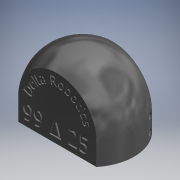
# Autodesk Inventor part: Wheel cover Alpha
Saved by Autodesk Inventor 2019 (Build 230136000, 136)
## iProperties
Part Number: Wheel cover Alpha
Material: Generic
Document SubType Name: Modeling
Designer: Delta
Appearance: Default
Author: Delta
Autodesk Inventor part; units mm, degrees
ref_plane "YZ Plane" through (0, 0, 0) normal (1, 0, 0) x (0, 1, 0)
ref_plane "XZ Plane" through (0, 0, 0) normal (0, 1, 0) x (-1, 0, 0)
ref_plane "XY Plane" through (0, 0, 0) normal (0, 0, 1) x (1, 0, 0)
sketch "Sketch1" plane through (0, 0, 0) normal (0, 0, 1) x (1, 0, 0)
  circle A0 centre (0, 0) radius 41.275
  circle A1 centre (0, 0) radius 44.45
  line L0 (-44.45, 0) -> (-41.275, 0)
  line L1 (41.275, 0) -> (44.45, 0)
  line L2 (-44.45, 0) -> (-41.275, 0)
  line L3 (-41.275, 0) -> (-41.275, -25.4)
  line L4 (-41.275, -25.4) -> (-44.45, -25.4)
  line L5 (-44.45, -25.4) -> (-44.45, 0)
  line L6 (41.275, 0) -> (44.45, 0)
  line L7 (44.45, 0) -> (44.45, -25.4)
  line L8 (44.45, -25.4) -> (41.275, -25.4)
  line L9 (41.275, -25.4) -> (41.275, 0)
  dimension "d0" = 82.55
  dimension "d1" = 88.9
  dimension "d2" = 25.4
  dimension "d3" = 25.4
  constraints: 20 end point, 4 parallel, 4 point on circle, 3 horizontal, 2 centre point, 2 coincident, 2 perpendicular, 2 point on line
  measures "d0" diameter of A0
  measures "d1" diameter of A1
  measures "d2" distance of L2.end L3.end
  measures "d3" distance of L6.end L7.end
extrude "Extrusion1" add sketch "Sketch1" along normal blind 59.69 contours A0 L0 A1 L1 | L1 A1 L9 | L3 A1 L0 | L7 L8 L9 A1 | A1 L3 L4 L5
sketch "Sketch2" plane through (0, 0, 59.69) normal (0, 0, 1) x (1, 0, 0)
  line L0 (-44.45, -25.4) -> (-41.275, -25.4) projected
  arc A0 (44.45, 0) -> (-44.45, 0) centre (0, 0) ccw projected
  line L1 (-44.45, -25.4) -> (44.45, -25.4)
  line L2 (44.45, -25.4) -> (44.45, 0)
  line L3 (44.45, 0) -> (-44.45, 0)
  line L4 (-44.45, 0) -> (-44.45, -25.4)
  line L5 (44.45, -25.4) -> (44.45, 0) projected
  arc A1 (44.45, 0) -> (-44.45, 0) centre (0, 0) ccw
  constraints: 8 end point, 2 parallel, 2 point on circle, 1 centre point, 1 horizontal, 1 perpendicular, 1 tangent
extrude "Extrusion2" add sketch "Sketch2" along normal blind 3.175
sketch "Sketch3" plane through (41.275, -25.4, 0) normal (-1, 0, 0) x (0, 0, 1)
  line L0 (0, 0) -> (59.69, 0) projected
  line L1 (0, 0) -> (12.7, 0)
  line L2 (12.7, 0) -> (12.7, 25.4)
  line L3 (12.7, 25.4) -> (0, 25.4)
  line L4 (0, 25.4) -> (0, 0)
  dimension "d8" = 12.7
  dimension "d9" = 25.4
  constraints: 8 end point, 2 parallel, 1 horizontal, 1 perpendicular
  measures "d8" distance of L3.end L2.end
  measures "d9" distance of L2.end L1.end
extrude "Extrusion3" add sketch "Sketch3" along normal blind 9.525
ref_plane "Work Plane1" through (0, -25.4, 0) normal (-1, 0, 0) x (0, 0, 1)
mirror "Mirror1" about plane through (0, -25.4, 0) normal (-1, 0, 0) of "Extrusion3"
ref_plane "Work Plane2" through (41.275, 0, 0) normal (0, -1, 0) x (1, 0, 0)
sketch "Sketch5" plane through (41.275, 0, 0) normal (0, -1, 0) x (1, 0, 0)
  line L0 (-85.725, 0) -> (-85.725, 62.865) projected
  line L1 (-85.725, 0) -> (-85.725, 62.865)
  arc A0 (-85.725, 62.865) -> (-85.725, 0) centre (-47.625, 31.4325) ccw
  line L2 (-41.275, 62.865) -> (-41.275, -18.3182)
  line L3 (3.175, 0) -> (3.175, 62.865) projected
  dimension "d12" = 44.45
  dimension "d13" = 44.45
  dimension "d33" = 38.1
  constraints: 4 end point, 2 point on circle, 2 vertical, 1 centre point
  measures "d12" distance between parallel lines of L3 L2
  measures "d13" distance between parallel lines of L0 L2
  measures "d33" distance from line of L0 A0.centre
revolve "Revolution1" add sketch "Sketch5" angle 180 about axis through (0, 0, 62.865) along (0, 0, -1)
sketch "Sketch6" plane through (6.35, 0, 31.4325) normal (0, -1, 0) x (1, 0, 0)
  line L0 (38.1, -31.4325) -> (38.1, 31.4325) projected
  line L1 (38.1, -31.4325) -> (38.1, 31.4325)
  arc A0 (38.1, -31.4325) -> (38.1, 31.4325) centre (0, 0) ccw projected
  line L2 (38.1, -31.4325) -> (38.1, 31.4325) projected
  arc A1 (38.1, -31.4325) -> (38.1, 31.4325) centre (0, 0) ccw
  point P0 (-6.35, -31.4325)
  constraints: 2 end point, 2 point on circle, 1 centre point, 1 collinear, 1 concentric
extrude "Extrusion4" add sketch "Sketch6" along normal blind 25.4
ref_plane "Work Plane3" through (0, -25.4, 0) normal (1, 0, 0) x (0, 0, -1)
mirror "Mirror2" about plane through (0, -25.4, 0) normal (1, 0, 0) of "Extrusion4"
sketch "Sketch7" plane through (31.75, -25.4, 0) normal (-1, 0, 0) x (0, 0, 1)
  line L0 (12.7, 0) -> (12.7, 25.4) projected
  line L1 (0, 25.4) -> (0, 0) projected
  line L2 (0, 0) -> (12.7, 0) projected
  circle A0 centre (6.35, 24.003) radius 1.524
  circle A1 centre (6.35, 8.001) radius 1.524
  dimension "d18" = 6.35
  dimension "d19" = 6.35
  dimension "d20" = 8.001
  dimension "d21" = 24.003
  dimension "d22" = 6.35
  dimension "d25" = 3.048
  dimension "d26" = 3.048
  constraints: 2 centre point, 2 coincident
  measures "d18" distance from line of L0 point (6.35, 8.001)
  measures "d19" distance from line of L1 point (6.35, 8.001)
  measures "d20" distance from line of L2 point (6.35, 8.001)
  measures "d21" distance from line of point (6.35, 24.003) L2
  measures "d22" distance from line of L0 point (6.35, 24.003)
  measures "d25" diameter of A0
  measures "d26" diameter of A1
sketch "Sketch8" plane through (31.75, 0, 0) normal (0, 1, 0) x (1, 0, 0)
  line L0 (9.525, -12.7) -> (9.525, -59.69) projected
  line L1 (0, -12.7) -> (0, 0) projected
  line L2 (9.525, -12.7) -> (0, -12.7)
  line L3 (0, -12.7) -> (0, 0)
  line L4 (0, 0) -> (9.525, 0)
  line L5 (9.525, 0) -> (9.525, -12.7)
  point P0 (-31.75, 0)
  constraints: 8 end point, 2 parallel, 1 horizontal, 1 perpendicular
extrude "Extrusion5" add sketch "Sketch8" along normal blind 2.54
extrude "Extrusion6" cut sketch "Sketch7" against normal through all
ref_plane "Work Plane4" through (55.7424, 0, 31.4325) normal (-1, 0, 0) x (0, -1, 0)
sketch "Sketch9" plane through (55.7424, 0, 31.4325) normal (-1, 0, 0) x (0, -1, 0)
  circle A0 centre (17.399, -25.0825) radius 1.524 projected
  circle A1 centre (17.399, -25.0825) radius 3.175
  circle A2 centre (1.397, -25.0825) radius 1.524 projected
  circle A3 centre (1.397, -25.0825) radius 3.175
  point P0 (0, -31.4325)
  dimension "d29" = 6.35
  dimension "d30" = 6.35
  constraints: 2 centre point, 2 coincident
  measures "d29" diameter of A1
  measures "d30" diameter of A3
extrude "Extrusion7" cut sketch "Sketch9" along normal blind 19.05
ref_plane "Work Plane5" through (0, -25.4, 0) normal (1, 0, 0) x (0, 0, -1)
mirror "Mirror3" about plane through (0, -25.4, 0) normal (1, 0, 0) of "Extrusion7", "Extrusion6", "Extrusion5"
sketch "Sketch10" plane through (0, 0, 59.69) normal (0, 0, -1) x (-1, 0, 0)
  line L0 (-11.0899, 12.4283) -> (34.7993, 12.4283) construction
  line L1 (34.7993, 12.4283) -> (34.7993, -9.7515) construction
  line L2 (34.7993, -9.7515) -> (-11.0899, -9.7515) construction
  line L3 (-11.0899, -9.7515) -> (-11.0899, 12.4283) construction
  line L4 (-4.0812, -3.8275) -> (-7.6627, -12.2101)
  line L5 (-7.6627, -12.2101) -> (-9.5307, -12.2101)
  line L6 (-9.5307, -12.2101) -> (-7.2768, -3.8275)
  line L7 (-7.2768, -3.8275) -> (-4.0812, -3.8275)
  line L8 (-4.9303, 3.1812) -> (-7.9869, 3.1812)
  line L9 (-7.9869, 3.1812) -> (-7.9869, 6.8245)
  line L10 (-7.9869, 6.8245) -> (-4.9303, 6.8245)
  line L11 (-4.9303, 6.8245) -> (-4.9303, 3.1812)
  spline S0 degree 2 poles (6.8332, -0.1533) (6.8332, -4.1053) (4.3014, -10.0951) (2.0629, -12.735) knots 0 0 0 1 2 2 2
  line L12 (2.0629, -12.735) -> (-0.8702, -12.735)
  line L13 (-0.8702, -12.735) -> (-0.8702, -12.6115)
  spline S1 degree 2 poles (-0.8702, -12.6115) (0.1178, -11.7315) (2.1093, -9.1534) (2.8503, -7.6097) knots 0 0 0 1 2 2 2
  spline S2 degree 2 poles (2.8503, -7.6097) (3.653, -5.9579) (4.5793, -2.2837) (4.5793, -0.1533) knots 0 0 0 1 2 2 2
  spline S3 degree 2 poles (4.5793, -0.1533) (4.5793, 1.9616) (3.6376, 5.713) (2.8503, 7.303) knots 0 0 0 1 2 2 2
  spline S4 degree 2 poles (2.8503, 7.303) (2.0784, 8.8931) (0.1024, 11.4249) (-0.8702, 12.3048) knots 0 0 0 1 2 2 2
  line L14 (-0.8702, 12.3048) -> (-0.8702, 12.4283)
  line L15 (-0.8702, 12.4283) -> (2.0629, 12.4283)
  spline S5 degree 2 poles (2.0629, 12.4283) (4.286, 9.7885) (6.8332, 3.8296) (6.8332, -0.1533) knots 0 0 0 1 2 2 2
  point P0 (0, 0)
  constraints: 2 other
extrude "Extrusion8" cut sketch "Sketch10" against normal blind 1.27
sketch "Sketch11" plane through (0, 0, 62.865) normal (0, 0, 1) x (1, 0, 0)
  line L0 (-39.7477, -3.175) -> (39.7477, -3.175) construction
  line L1 (39.7477, -3.175) -> (39.7477, -22.225) construction
  line L2 (39.7477, -22.225) -> (-39.7477, -22.225) construction
  line L3 (-39.7477, -22.225) -> (-39.7477, -3.175) construction
  line L4 (-42.9227, -25.4) -> (-42.9227, 0) projected
  line L5 (42.9227, 0) -> (42.9227, -25.4) projected
  line L6 (-44.45, -25.4) -> (44.45, -25.4) projected
  arc A0 (42.9227, 0) -> (-42.9227, 0) centre (0, 0) ccw projected
  line L7 (42.9227, -25.4) -> (42.9227, 0) projected
  line L8 (-42.9227, 0) -> (42.9227, 0)
  line L9 (0, 0) -> (0, 42.9227)
  arc A1 (30.2227, 0) -> (-30.2227, 0) centre (0, 0) ccw
  spline S0 degree 2 poles (-39.0273, -8.6682) (-39.0273, -7.4461) (-38.2297, -5.4135) (-37.535, -4.6802) knots 0 0 0 1 2 2 2
  spline S1 degree 2 poles (-37.535, -4.6802) (-36.8789, -3.9726) (-34.9621, -3.1879) (-33.9844, -3.1879) knots 0 0 0 1 2 2 2
  spline S2 degree 2 poles (-33.9844, -3.1879) (-32.8909, -3.1879) (-31.1155, -3.9212) (-30.4594, -4.6158) knots 0 0 0 1 2 2 2
  spline S3 degree 2 poles (-30.4594, -4.6158) (-29.6361, -5.4906) (-28.7356, -8.3209) (-28.7356, -10.495) knots 0 0 0 1 2 2 2
  spline S4 degree 2 poles (-28.7356, -10.495) (-28.7356, -12.4633) (-29.6232, -15.9882) (-30.4852, -17.1589) knots 0 0 0 1 2 2 2
  spline S5 degree 2 poles (-30.4852, -17.1589) (-31.3986, -18.3939) (-33.9715, -19.6932) (-35.8497, -19.6932) knots 0 0 0 1 2 2 2
  spline S6 degree 2 poles (-35.8497, -19.6932) (-36.2743, -19.6932) (-37.2391, -19.6032) (-37.6508, -19.4745) knots 0 0 0 1 2 2 2
  line L10 (-37.6508, -19.4745) -> (-37.6508, -17.4291)
  line L11 (-37.6508, -17.4291) -> (-37.5479, -17.4291)
  spline S7 degree 2 poles (-37.5479, -17.4291) (-37.2777, -17.5834) (-36.1456, -17.8536) (-35.5667, -17.8536) knots 0 0 0 1 2 2 2
  spline S8 degree 2 poles (-35.5667, -17.8536) (-33.4826, -17.8536) (-31.1027, -15.1005) (-30.9354, -12.5533) knots 0 0 0 1 2 2 2
  spline S9 degree 2 poles (-30.9354, -12.5533) (-31.7845, -13.1323) (-33.3283, -13.6597) (-34.2417, -13.6597) knots 0 0 0 1 2 2 2
  spline S10 degree 2 poles (-34.2417, -13.6597) (-35.1164, -13.6597) (-36.5702, -13.2738) (-37.3034, -12.7206) knots 0 0 0 1 2 2 2
  spline S11 degree 2 poles (-37.3034, -12.7206) (-38.1525, -12.0645) (-39.0273, -10.0705) (-39.0273, -8.6682) knots 0 0 0 1 2 2 2
  spline S12 degree 2 poles (-30.884, -10.019) (-30.884, -8.4109) (-31.4757, -6.3783) (-32.0032, -5.8251) knots 0 0 0 1 2 2 2
  spline S13 degree 2 poles (-32.0032, -5.8251) (-32.4663, -5.3105) (-33.4312, -4.9246) (-33.9972, -4.9246) knots 0 0 0 1 2 2 2
  spline S14 degree 2 poles (-33.9972, -4.9246) (-35.3094, -4.9246) (-36.866, -6.8028) (-36.866, -8.5782) knots 0 0 0 1 2 2 2
  spline S15 degree 2 poles (-36.866, -8.5782) (-36.866, -9.5816) (-36.3515, -10.8809) (-35.7854, -11.3441) knots 0 0 0 1 2 2 2
  spline S16 degree 2 poles (-35.7854, -11.3441) (-35.3737, -11.6785) (-34.3574, -11.8972) (-33.7657, -11.8972) knots 0 0 0 1 2 2 2
  spline S17 degree 2 poles (-33.7657, -11.8972) (-33.0838, -11.8972) (-31.5143, -11.4213) (-30.9226, -11.0224) knots 0 0 0 1 2 2 2
  spline S18 degree 2 poles (-30.9226, -11.0224) (-30.9097, -10.8681) (-30.884, -10.3406) (-30.884, -10.019) knots 0 0 0 1 2 2 2
  spline S19 degree 2 poles (-27.1146, -8.6682) (-27.1146, -7.4461) (-26.317, -5.4135) (-25.6223, -4.6802) knots 0 0 0 1 2 2 2
  spline S20 degree 2 poles (-25.6223, -4.6802) (-24.9662, -3.9726) (-23.0494, -3.1879) (-22.0717, -3.1879) knots 0 0 0 1 2 2 2
  spline S21 degree 2 poles (-22.0717, -3.1879) (-20.9782, -3.1879) (-19.2029, -3.9212) (-18.5468, -4.6158) knots 0 0 0 1 2 2 2
  spline S22 degree 2 poles (-18.5468, -4.6158) (-17.7234, -5.4906) (-16.8229, -8.3209) (-16.8229, -10.495) knots 0 0 0 1 2 2 2
  spline S23 degree 2 poles (-16.8229, -10.495) (-16.8229, -12.4633) (-17.7106, -15.9882) (-18.5725, -17.1589) knots 0 0 0 1 2 2 2
  spline S24 degree 2 poles (-18.5725, -17.1589) (-19.4859, -18.3939) (-22.0588, -19.6932) (-23.9371, -19.6932) knots 0 0 0 1 2 2 2
  spline S25 degree 2 poles (-23.9371, -19.6932) (-24.3616, -19.6932) (-25.3264, -19.6032) (-25.7381, -19.4745) knots 0 0 0 1 2 2 2
  line L12 (-25.7381, -19.4745) -> (-25.7381, -17.4291)
  line L13 (-25.7381, -17.4291) -> (-25.6352, -17.4291)
  spline S26 degree 2 poles (-25.6352, -17.4291) (-25.365, -17.5834) (-24.2329, -17.8536) (-23.654, -17.8536) knots 0 0 0 1 2 2 2
  spline S27 degree 2 poles (-23.654, -17.8536) (-21.57, -17.8536) (-19.19, -15.1005) (-19.0227, -12.5533) knots 0 0 0 1 2 2 2
  spline S28 degree 2 poles (-19.0227, -12.5533) (-19.8718, -13.1323) (-21.4156, -13.6597) (-22.329, -13.6597) knots 0 0 0 1 2 2 2
  spline S29 degree 2 poles (-22.329, -13.6597) (-23.2038, -13.6597) (-24.6575, -13.2738) (-25.3908, -12.7206) knots 0 0 0 1 2 2 2
  spline S30 degree 2 poles (-25.3908, -12.7206) (-26.2398, -12.0645) (-27.1146, -10.0705) (-27.1146, -8.6682) knots 0 0 0 1 2 2 2
  spline S31 degree 2 poles (-18.9713, -10.019) (-18.9713, -8.4109) (-19.5631, -6.3783) (-20.0905, -5.8251) knots 0 0 0 1 2 2 2
  spline S32 degree 2 poles (-20.0905, -5.8251) (-20.5536, -5.3105) (-21.5185, -4.9246) (-22.0845, -4.9246) knots 0 0 0 1 2 2 2
  spline S33 degree 2 poles (-22.0845, -4.9246) (-23.3967, -4.9246) (-24.9534, -6.8028) (-24.9534, -8.5782) knots 0 0 0 1 2 2 2
  spline S34 degree 2 poles (-24.9534, -8.5782) (-24.9534, -9.5816) (-24.4388, -10.8809) (-23.8727, -11.3441) knots 0 0 0 1 2 2 2
  spline S35 degree 2 poles (-23.8727, -11.3441) (-23.4611, -11.6785) (-22.4448, -11.8972) (-21.853, -11.8972) knots 0 0 0 1 2 2 2
  spline S36 degree 2 poles (-21.853, -11.8972) (-21.1711, -11.8972) (-19.6017, -11.4213) (-19.0099, -11.0224) knots 0 0 0 1 2 2 2
  spline S37 degree 2 poles (-19.0099, -11.0224) (-18.997, -10.8681) (-18.9713, -10.3406) (-18.9713, -10.019) knots 0 0 0 1 2 2 2
  line L14 (4.5196, -19.3845) -> (-9.207, -19.3845)
  line L15 (-9.207, -19.3845) -> (-3.6495, -3.5095)
  line L16 (-3.6495, -3.5095) -> (-1.0379, -3.5095)
  line L17 (-1.0379, -3.5095) -> (4.5196, -19.3845)
  line L18 (1.6765, -17.5577) -> (-2.4016, -5.5936)
  line L19 (-2.4016, -5.5936) -> (-6.454, -17.5577)
  line L20 (-6.454, -17.5577) -> (1.6765, -17.5577)
  line L21 (22.3886, -19.3845) -> (12.5986, -19.3845)
  line L22 (12.5986, -19.3845) -> (12.5986, -17.1332)
  spline S38 degree 2 poles (12.5986, -17.1332) (13.6535, -16.1426) (15.5317, -14.3029) (16.4323, -13.3124) knots 0 0 0 1 2 2 2
  spline S39 degree 2 poles (16.4323, -13.3124) (18.2462, -11.3183) (19.5713, -8.9255) (19.5713, -7.6519) knots 0 0 0 1 2 2 2
  spline S40 degree 2 poles (19.5713, -7.6519) (19.5713, -6.9829) (19.1596, -5.9795) (18.7865, -5.6579) knots 0 0 0 1 2 2 2
  spline S41 degree 2 poles (18.7865, -5.6579) (18.4134, -5.3363) (17.4357, -5.0146) (16.8439, -5.0146) knots 0 0 0 1 2 2 2
  spline S42 degree 2 poles (16.8439, -5.0146) (16.2779, -5.0146) (15.1201, -5.2977) (14.5926, -5.5164) knots 0 0 0 1 2 2 2
  spline S43 degree 2 poles (14.5926, -5.5164) (14.1424, -5.6965) (13.3062, -6.2111) (13.0489, -6.3912) knots 0 0 0 1 2 2 2
  line L23 (13.0489, -6.3912) -> (12.9331, -6.3912)
  line L24 (12.9331, -6.3912) -> (12.9331, -4.127)
  spline S44 degree 2 poles (12.9331, -4.127) (13.5892, -3.8054) (15.9434, -3.175) (16.9983, -3.175) knots 0 0 0 1 2 2 2
  spline S45 degree 2 poles (16.9983, -3.175) (19.2239, -3.175) (21.7325, -5.5292) (21.7325, -7.5361) knots 0 0 0 1 2 2 2
  spline S46 degree 2 poles (21.7325, -7.5361) (21.7325, -8.4752) (21.2951, -10.0447) (20.9092, -10.7137) knots 0 0 0 1 2 2 2
  spline S47 degree 2 poles (20.9092, -10.7137) (20.5232, -11.4084) (19.404, -12.772) (18.7865, -13.4281) knots 0 0 0 1 2 2 2
  spline S48 degree 2 poles (18.7865, -13.4281) (17.7831, -14.5216) (15.3259, -16.863) (14.5926, -17.5448) knots 0 0 0 1 2 2 2
  line L25 (14.5926, -17.5448) -> (22.3886, -17.5448)
  line L26 (22.3886, -17.5448) -> (22.3886, -19.3845)
  spline S49 degree 2 poles (34.1341, -14.3415) (34.1341, -15.4865) (33.4008, -17.4419) (32.7318, -18.1623) knots 0 0 0 1 2 2 2
  spline S50 degree 2 poles (32.7318, -18.1623) (32.0628, -18.8828) (30.0688, -19.719) (28.8338, -19.719) knots 0 0 0 1 2 2 2
  spline S51 degree 2 poles (28.8338, -19.719) (27.7017, -19.719) (25.489, -19.2172) (24.6785, -18.8184) knots 0 0 0 1 2 2 2
  line L27 (24.6785, -18.8184) -> (24.6785, -16.5671)
  line L28 (24.6785, -16.5671) -> (24.8329, -16.5671)
  spline S52 degree 2 poles (24.8329, -16.5671) (25.0773, -16.7472) (25.9907, -17.2104) (26.5439, -17.4162) knots 0 0 0 1 2 2 2
  spline S53 degree 2 poles (26.5439, -17.4162) (27.1743, -17.6349) (28.2163, -17.8793) (28.8724, -17.8793) knots 0 0 0 1 2 2 2
  spline S54 degree 2 poles (28.8724, -17.8793) (29.5156, -17.8793) (30.7249, -17.4162) (31.1623, -16.9145) knots 0 0 0 1 2 2 2
  spline S55 degree 2 poles (31.1623, -16.9145) (31.5611, -16.4385) (31.9728, -15.1777) (31.9728, -14.3287) knots 0 0 0 1 2 2 2
  spline S56 degree 2 poles (31.9728, -14.3287) (31.9728, -13.4796) (31.5097, -12.399) (31.0723, -12.0388) knots 0 0 0 1 2 2 2
  spline S57 degree 2 poles (31.0723, -12.0388) (30.622, -11.64) (29.2841, -11.3055) (28.4736, -11.3055) knots 0 0 0 1 2 2 2
  spline S58 degree 2 poles (28.4736, -11.3055) (27.5988, -11.3055) (25.8621, -11.5756) (25.3346, -11.6914) knots 0 0 0 1 2 2 2
  line L29 (25.3346, -11.6914) -> (25.3346, -3.5095)
  line L30 (25.3346, -3.5095) -> (34.044, -3.5095)
  line L31 (34.044, -3.5095) -> (34.044, -5.3749)
  line L32 (34.044, -5.3749) -> (27.3801, -5.3749)
  line L33 (27.3801, -5.3749) -> (27.3801, -9.6073)
  spline S59 degree 2 poles (27.3801, -9.6073) (27.766, -9.5559) (28.5122, -9.5173) (28.8209, -9.5173) knots 0 0 0 1 2 2 2
  spline S60 degree 2 poles (28.8209, -9.5173) (30.0431, -9.5173) (31.7284, -9.9161) (32.5002, -10.5079) knots 0 0 0 1 2 2 2
  spline S61 degree 2 poles (32.5002, -10.5079) (33.285, -11.0996) (34.1341, -12.9007) (34.1341, -14.3415) knots 0 0 0 1 2 2 2
  spline S62 degree 2 poles (-31.9263, 14.8461) (-30.6882, 14.4351) (-29.0287, 12.7701) (-28.7516, 11.7429) knots 0 0 0 1 2 2 2
  spline S63 degree 2 poles (-28.7516, 11.7429) (-28.5479, 10.9108) (-28.7241, 9.3996) (-29.0889, 8.3008) knots 0 0 0 1 2 2 2
  line L34 (-29.0889, 8.3008) -> (-29.7794, 6.2202)
  line L35 (-29.7794, 6.2202) -> (-38.8195, 9.2207)
  line L36 (-38.8195, 9.2207) -> (-38.1362, 11.2793)
  spline S64 degree 2 poles (-38.1362, 11.2793) (-37.7131, 12.554) (-36.8508, 13.878) (-36.3436, 14.279) knots 0 0 0 1 2 2 2
  spline S65 degree 2 poles (-36.3436, 14.279) (-35.4755, 14.9587) (-33.2449, 15.2837) (-31.9263, 14.8461) knots 0 0 0 1 2 2 2
  spline S66 degree 2 poles (-32.3567, 13.5982) (-33.397, 13.9435) (-35.098, 13.7436) (-35.7417, 13.2009) knots 0 0 0 1 2 2 2
  spline S67 degree 2 poles (-35.7417, 13.2009) (-36.1879, 12.8122) (-36.8066, 11.8058) (-37.0765, 10.9926) knots 0 0 0 1 2 2 2
  line L37 (-37.0765, 10.9926) -> (-37.3804, 10.0769)
  line L38 (-37.3804, 10.0769) -> (-30.4209, 7.7669)
  line L39 (-30.4209, 7.7669) -> (-30.117, 8.6827)
  spline S68 degree 2 poles (-30.117, 8.6827) (-29.8519, 9.4812) (-29.7071, 10.775) (-29.8885, 11.3802) knots 0 0 0 1 2 2 2
  spline S69 degree 2 poles (-29.8885, 11.3802) (-30.1043, 12.1512) (-31.3018, 13.2481) (-32.3567, 13.5982) knots 0 0 0 1 2 2 2
  spline S70 degree 2 poles (-24.8557, 16.915) (-25.7947, 15.4816) (-28.4345, 14.9594) (-29.9195, 15.9322) knots 0 0 0 1 2 2 2
  spline S71 degree 2 poles (-29.9195, 15.9322) (-31.3787, 16.8881) (-32.1067, 19.5519) (-31.2988, 20.7852) knots 0 0 0 1 2 2 2
  spline S72 degree 2 poles (-31.2988, 20.7852) (-30.935, 21.3404) (-30.0496, 21.9877) (-29.5002, 22.0799) knots 0 0 0 1 2 2 2
  spline S73 degree 2 poles (-29.5002, 22.0799) (-28.9465, 22.1786) (-27.7344, 21.8736) (-27.0177, 21.4041) knots 0 0 0 1 2 2 2
  line L40 (-27.0177, 21.4041) -> (-26.4689, 21.0446)
  line L41 (-26.4689, 21.0446) -> (-29.1802, 16.9058)
  spline S74 degree 2 poles (-29.1802, 16.9058) (-28.1407, 16.2248) (-26.3513, 16.5475) (-25.7423, 17.4773) knots 0 0 0 1 2 2 2
  spline S75 degree 2 poles (-25.7423, 17.4773) (-25.5265, 17.8066) (-25.2563, 18.5431) (-25.2033, 18.8775) knots 0 0 0 1 2 2 2
  spline S76 degree 2 poles (-25.2033, 18.8775) (-25.1548, 19.2333) (-25.1355, 19.7558) (-25.1584, 19.9462) knots 0 0 0 1 2 2 2
  line L42 (-25.1584, 19.9462) -> (-25.1203, 20.0043)
  line L43 (-25.1203, 20.0043) -> (-24.0227, 19.2852)
  spline S77 degree 2 poles (-24.0227, 19.2852) (-24.0659, 19.0643) (-24.2061, 18.3995) (-24.2834, 18.1549) knots 0 0 0 1 2 2 2
  spline S78 degree 2 poles (-24.2834, 18.1549) (-24.3898, 17.8093) (-24.6188, 17.2765) (-24.8557, 16.915) knots 0 0 0 1 2 2 2
  spline S79 degree 2 poles (-27.8802, 20.5665) (-28.2954, 20.8201) (-28.9994, 21.0413) (-29.3053, 21.011) knots 0 0 0 1 2 2 2
  spline S80 degree 2 poles (-29.3053, 21.011) (-29.6455, 20.9847) (-30.2439, 20.5924) (-30.5104, 20.1856) knots 0 0 0 1 2 2 2
  spline S81 degree 2 poles (-30.5104, 20.1856) (-30.7726, 19.7853) (-30.9017, 19.0671) (-30.8216, 18.6824) knots 0 0 0 1 2 2 2
  spline S82 degree 2 poles (-30.8216, 18.6824) (-30.7307, 18.2999) (-30.3083, 17.691) (-29.9485, 17.4092) knots 0 0 0 1 2 2 2
  line L44 (-29.9485, 17.4092) -> (-27.8802, 20.5665)
  line L45 (-21.85, 20.8891) -> (-22.6646, 20.0023)
  line L46 (-22.6646, 20.0023) -> (-29.9918, 26.7332)
  line L47 (-29.9918, 26.7332) -> (-29.1772, 27.62)
  line L48 (-29.1772, 27.62) -> (-21.85, 20.8891)
  spline S83 degree 2 poles (-18.8752, 23.4407) (-19.6213, 22.8048) (-21.1874, 22.9405) (-21.9735, 23.8628) knots 0 0 0 1 2 2 2
  line L49 (-21.9735, 23.8628) -> (-24.5422, 26.8763)
  line L50 (-24.5422, 26.8763) -> (-25.159, 26.3506)
  line L51 (-25.159, 26.3506) -> (-25.8049, 27.1084)
  line L52 (-25.8049, 27.1084) -> (-25.1881, 27.6341)
  line L53 (-25.1881, 27.6341) -> (-26.5201, 29.1967)
  line L54 (-26.5201, 29.1967) -> (-25.6037, 29.9778)
  line L55 (-25.6037, 29.9778) -> (-24.2717, 28.4152)
  line L56 (-24.2717, 28.4152) -> (-22.5858, 29.8523)
  line L57 (-22.5858, 29.8523) -> (-21.9399, 29.0945)
  line L58 (-21.9399, 29.0945) -> (-23.6258, 27.6575)
  line L59 (-23.6258, 27.6575) -> (-21.4176, 25.0669)
  spline S84 degree 2 poles (-21.4176, 25.0669) (-21.0671, 24.6557) (-20.6522, 24.2284) (-20.3871, 24.1197) knots 0 0 0 1 2 2 2
  spline S85 degree 2 poles (-20.3871, 24.1197) (-20.1596, 24.0194) (-19.6443, 24.1645) (-19.3271, 24.4349) knots 0 0 0 1 2 2 2
  spline S86 degree 2 poles (-19.3271, 24.4349) (-19.1039, 24.6252) (-18.802, 25.1158) (-18.7431, 25.237) knots 0 0 0 1 2 2 2
  line L60 (-18.7431, 25.237) -> (-18.6902, 25.2821)
  line L61 (-18.6902, 25.2821) -> (-17.9892, 24.4597)
  spline S87 degree 2 poles (-17.9892, 24.4597) (-18.1876, 24.1689) (-18.6461, 23.636) (-18.8752, 23.4407) knots 0 0 0 1 2 2 2
  spline S88 degree 2 poles (-14.1689, 27.5855) (-14.2424, 27.4188) (-14.4792, 26.8384) (-14.6226, 26.6228) knots 0 0 0 1 2 2 2
  spline S89 degree 2 poles (-14.6226, 26.6228) (-14.8128, 26.3182) (-15.2403, 25.8687) (-15.7092, 25.6001) knots 0 0 0 1 2 2 2
  spline S90 degree 2 poles (-15.7092, 25.6001) (-16.0909, 25.3815) (-16.9458, 25.2743) (-17.3566, 25.3859) knots 0 0 0 1 2 2 2
  spline S91 degree 2 poles (-17.3566, 25.3859) (-17.7502, 25.4985) (-18.4813, 26.076) (-18.7192, 26.4912) knots 0 0 0 1 2 2 2
  spline S92 degree 2 poles (-18.7192, 26.4912) (-19.0875, 27.1342) (-19.0668, 28.3559) (-18.627, 28.9547) knots 0 0 0 1 2 2 2
  spline S93 degree 2 poles (-18.627, 28.9547) (-18.2427, 29.4951) (-16.9263, 30.4893) (-16.1293, 31.0081) knots 0 0 0 1 2 2 2
  line L62 (-16.1293, 31.0081) -> (-16.2444, 31.209)
  spline S94 degree 2 poles (-16.2444, 31.209) (-16.4516, 31.5707) (-16.9297, 31.8928) (-17.2035, 31.905) knots 0 0 0 1 2 2 2
  spline S95 degree 2 poles (-17.2035, 31.905) (-17.4773, 31.9171) (-18.0994, 31.6676) (-18.4075, 31.4911) knots 0 0 0 1 2 2 2
  spline S96 degree 2 poles (-18.4075, 31.4911) (-18.7692, 31.2839) (-19.6243, 30.5095) (-19.9943, 30.0218) knots 0 0 0 1 2 2 2
  line L63 (-19.9943, 30.0218) -> (-20.0546, 29.9872)
  line L64 (-20.0546, 29.9872) -> (-20.6646, 31.0522)
  spline S97 degree 2 poles (-20.6646, 31.0522) (-20.4226, 31.2975) (-19.4594, 32.1161) (-18.9302, 32.4192) knots 0 0 0 1 2 2 2
  spline S98 degree 2 poles (-18.9302, 32.4192) (-18.2873, 32.7875) (-17.2947, 33.0892) (-16.7968, 33.0275) knots 0 0 0 1 2 2 2
  spline S99 degree 2 poles (-16.7968, 33.0275) (-16.3095, 32.9686) (-15.5103, 32.35) (-15.1766, 31.7673) knots 0 0 0 1 2 2 2
  line L65 (-15.1766, 31.7673) -> (-12.748, 27.5276)
  line L66 (-12.748, 27.5276) -> (-13.7929, 26.9291)
  line L67 (-13.7929, 26.9291) -> (-14.1689, 27.5855)
  line L68 (-14.6676, 28.4562) -> (-15.6536, 30.1775)
  spline S100 degree 2 poles (-15.6536, 30.1775) (-16.0095, 29.9292) (-17.0762, 29.167) (-17.3698, 28.8565) knots 0 0 0 1 2 2 2
  spline S101 degree 2 poles (-17.3698, 28.8565) (-17.7122, 28.4913) (-17.9516, 27.6514) (-17.6831, 27.1826) knots 0 0 0 1 2 2 2
  spline S102 degree 2 poles (-17.6831, 27.1826) (-17.3761, 26.6468) (-16.4626, 26.4495) (-15.8866, 26.7795) knots 0 0 0 1 2 2 2
  spline S103 degree 2 poles (-15.8866, 26.7795) (-15.3976, 27.0595) (-14.8356, 27.9419) (-14.6676, 28.4562) knots 0 0 0 1 2 2 2
  line L69 (0.072, 30.5231) -> (-1.5565, 30.2968)
  line L70 (-1.5565, 30.2968) -> (-5.0598, 33.6364)
  line L71 (-5.0598, 33.6364) -> (-6.4971, 33.4366)
  line L72 (-6.4971, 33.4366) -> (-5.9755, 29.6828)
  line L73 (-5.9755, 29.6828) -> (-7.2293, 29.5086)
  line L74 (-7.2293, 29.5086) -> (-8.5403, 38.9429)
  line L75 (-8.5403, 38.9429) -> (-6.1091, 39.2807)
  spline S104 degree 2 poles (-6.1091, 39.2807) (-5.2987, 39.3934) (-4.1809, 39.3694) (-3.6394, 39.1174) knots 0 0 0 1 2 2 2
  spline S105 degree 2 poles (-3.6394, 39.1174) (-3.0978, 38.8653) (-2.3852, 37.9435) (-2.2822, 37.2019) knots 0 0 0 1 2 2 2
  spline S106 degree 2 poles (-2.2822, 37.2019) (-2.1388, 36.1697) (-2.9994, 34.624) (-3.8548, 34.1623) knots 0 0 0 1 2 2 2
  line L76 (-3.8548, 34.1623) -> (0.072, 30.5231)
  spline S107 degree 2 poles (-3.5757, 36.9208) (-3.6331, 37.3337) (-4.0118, 37.9279) (-4.3463, 38.0918) knots 0 0 0 1 2 2 2
  spline S108 degree 2 poles (-4.3463, 38.0918) (-4.6383, 38.2304) (-5.3695, 38.2769) (-5.8894, 38.2047) knots 0 0 0 1 2 2 2
  line L77 (-5.8894, 38.2047) -> (-7.1356, 38.0315)
  line L78 (-7.1356, 38.0315) -> (-6.6426, 34.4841)
  line L79 (-6.6426, 34.4841) -> (-5.5417, 34.637)
  spline S109 degree 2 poles (-5.5417, 34.637) (-4.9989, 34.7125) (-4.1615, 35.0237) (-3.9048, 35.3633) knots 0 0 0 1 2 2 2
  spline S110 degree 2 poles (-3.9048, 35.3633) (-3.6657, 35.6614) (-3.5077, 36.4315) (-3.5757, 36.9208) knots 0 0 0 1 2 2 2
  spline S111 degree 2 poles (6.9711, 33.2234) (6.768, 31.4287) (4.821, 29.6681) (3.3791, 29.8313) knots 0 0 0 1 2 2 2
  spline S112 degree 2 poles (3.3791, 29.8313) (1.8988, 29.9988) (0.432, 32.2077) (0.6281, 33.9411) knots 0 0 0 1 2 2 2
  spline S113 degree 2 poles (0.6281, 33.9411) (0.8294, 35.7205) (2.8012, 37.4938) (4.2278, 37.3324) knots 0 0 0 1 2 2 2
  spline S114 degree 2 poles (4.2278, 37.3324) (5.6697, 37.1693) (7.1733, 35.0105) (6.9711, 33.2234) knots 0 0 0 1 2 2 2
  spline S115 degree 2 poles (5.7362, 33.3631) (5.8924, 34.7437) (5.0396, 36.1996) (4.1115, 36.3046) knots 0 0 0 1 2 2 2
  spline S116 degree 2 poles (4.1115, 36.3046) (3.1835, 36.4096) (2.0192, 35.182) (1.863, 33.8014) knots 0 0 0 1 2 2 2
  spline S117 degree 2 poles (1.863, 33.8014) (1.7111, 32.4592) (2.5673, 30.964) (3.4954, 30.859) knots 0 0 0 1 2 2 2
  spline S118 degree 2 poles (3.4954, 30.859) (4.4158, 30.7549) (5.5818, 31.9979) (5.7362, 33.3631) knots 0 0 0 1 2 2 2
  spline S119 degree 2 poles (14.6415, 30.7601) (14.0424, 29.1135) (11.7156, 27.6848) (10.5115, 28.1229) knots 0 0 0 1 2 2 2
  spline S120 degree 2 poles (10.5115, 28.1229) (9.9675, 28.3209) (9.289, 28.8717) (8.9963, 29.241) knots 0 0 0 1 2 2 2
  line L80 (8.9963, 29.241) -> (8.8102, 28.9555)
  line L81 (8.8102, 28.9555) -> (7.7512, 29.3408)
  line L82 (7.7512, 29.3408) -> (11.1531, 38.6907)
  line L83 (11.1531, 38.6907) -> (12.2846, 38.279)
  line L84 (12.2846, 38.279) -> (11.0706, 34.9423)
  spline S121 degree 2 poles (11.0706, 34.9423) (11.6385, 35.1711) (12.8169, 35.3173) (13.448, 35.0877) knots 0 0 0 1 2 2 2
  spline S122 degree 2 poles (13.448, 35.0877) (14.5868, 34.6733) (15.23, 32.3776) (14.6415, 30.7601) knots 0 0 0 1 2 2 2
  spline S123 degree 2 poles (13.442, 31.0979) (13.8801, 32.302) (13.6014, 33.8162) (12.789, 34.1118) knots 0 0 0 1 2 2 2
  spline S124 degree 2 poles (12.789, 34.1118) (12.3321, 34.278) (11.2307, 34.1859) (10.7249, 33.9921) knots 0 0 0 1 2 2 2
  line L85 (10.7249, 33.9921) -> (9.3235, 30.1405)
  spline S125 degree 2 poles (9.3235, 30.1405) (9.6749, 29.7744) (10.2717, 29.3601) (10.6634, 29.2176) knots 0 0 0 1 2 2 2
  spline S126 degree 2 poles (10.6634, 29.2176) (11.5265, 28.9036) (12.9591, 29.7705) (13.442, 31.0979) knots 0 0 0 1 2 2 2
  spline S127 degree 2 poles (21.3296, 26.4091) (20.3319, 24.9035) (17.7969, 24.2221) (16.5873, 25.0237) knots 0 0 0 1 2 2 2
  spline S128 degree 2 poles (16.5873, 25.0237) (15.3455, 25.8466) (15.0449, 28.4811) (16.0085, 29.9353) knots 0 0 0 1 2 2 2
  spline S129 degree 2 poles (16.0085, 29.9353) (16.9977, 31.428) (19.5605, 32.1095) (20.7573, 31.3164) knots 0 0 0 1 2 2 2
  spline S130 degree 2 poles (20.7573, 31.3164) (21.9669, 30.5148) (22.3231, 27.9083) (21.3296, 26.4091) knots 0 0 0 1 2 2 2
  spline S131 degree 2 poles (20.2937, 27.0956) (21.0612, 28.2537) (20.9645, 29.9383) (20.1859, 30.4542) knots 0 0 0 1 2 2 2
  spline S132 degree 2 poles (20.1859, 30.4542) (19.4074, 30.9701) (17.8119, 30.407) (17.0444, 29.2488) knots 0 0 0 1 2 2 2
  spline S133 degree 2 poles (17.0444, 29.2488) (16.2983, 28.1228) (16.3801, 26.4018) (17.1586, 25.8859) knots 0 0 0 1 2 2 2
  spline S134 degree 2 poles (17.1586, 25.8859) (17.9307, 25.3742) (19.5348, 25.9503) (20.2937, 27.0956) knots 0 0 0 1 2 2 2
  spline S135 degree 2 poles (21.6452, 20.91) (20.9447, 21.5957) (20.9388, 23.1676) (21.7865, 24.0336) knots 0 0 0 1 2 2 2
  line L86 (21.7865, 24.0336) -> (24.5564, 26.8634)
  line L87 (24.5564, 26.8634) -> (23.9772, 27.4303)
  line L88 (23.9772, 27.4303) -> (24.6737, 28.1419)
  line L89 (24.6737, 28.1419) -> (25.2529, 27.5749)
  line L90 (25.2529, 27.5749) -> (26.6892, 29.0422)
  line L91 (26.6892, 29.0422) -> (27.5497, 28.1999)
  line L92 (27.5497, 28.1999) -> (26.1134, 26.7326)
  line L93 (26.1134, 26.7326) -> (27.6965, 25.183)
  line L94 (27.6965, 25.183) -> (27, 24.4714)
  line L95 (27, 24.4714) -> (25.4169, 26.0211)
  line L96 (25.4169, 26.0211) -> (23.0358, 23.5885)
  spline S136 degree 2 poles (23.0358, 23.5885) (22.6578, 23.2024) (22.2696, 22.7506) (22.1852, 22.4768) knots 0 0 0 1 2 2 2
  spline S137 degree 2 poles (22.1852, 22.4768) (22.1059, 22.2413) (22.2968, 21.7411) (22.5947, 21.4496) knots 0 0 0 1 2 2 2
  spline S138 degree 2 poles (22.5947, 21.4496) (22.8043, 21.2444) (23.3201, 20.9879) (23.4461, 20.9401) knots 0 0 0 1 2 2 2
  line L97 (23.4461, 20.9401) -> (23.4958, 20.8915)
  line L98 (23.4958, 20.8915) -> (22.7399, 20.1193)
  spline S139 degree 2 poles (22.7399, 20.1193) (22.4324, 20.2907) (21.8603, 20.6994) (21.6452, 20.91) knots 0 0 0 1 2 2 2
  line L99 (23.9866, 18.3961) -> (23.2349, 19.3368)
  line L100 (23.2349, 19.3368) -> (28.8188, 23.7987)
  line L101 (28.8188, 23.7987) -> (29.5705, 22.858)
  line L102 (29.5705, 22.858) -> (23.9866, 18.3961)
  line L103 (30.5522, 23.5337) -> (29.6993, 24.6011)
  line L104 (29.6993, 24.6011) -> (30.6762, 25.3817)
  line L105 (30.6762, 25.3817) -> (31.529, 24.3143)
  line L106 (31.529, 24.3143) -> (30.5522, 23.5337)
  spline S140 degree 2 poles (26.3584, 14.4691) (25.9869, 15.1103) (25.7659, 16.4006) (25.9461, 17.0135) knots 0 0 0 1 2 2 2
  spline S141 degree 2 poles (25.9461, 17.0135) (26.1197, 17.6224) (27.0916, 18.7473) (27.9064, 19.2193) knots 0 0 0 1 2 2 2
  spline S142 degree 2 poles (27.9064, 19.2193) (28.7213, 19.6913) (30.1617, 19.9458) (30.7752, 19.8106) knots 0 0 0 1 2 2 2
  spline S143 degree 2 poles (30.7752, 19.8106) (31.3954, 19.6792) (32.4602, 18.842) (32.8239, 18.2141) knots 0 0 0 1 2 2 2
  spline S144 degree 2 poles (32.8239, 18.2141) (33.1179, 17.7065) (33.3801, 16.5917) (33.4058, 16.116) knots 0 0 0 1 2 2 2
  line L107 (33.4058, 16.116) -> (32.2369, 15.439)
  line L108 (32.2369, 15.439) -> (32.2021, 15.4991)
  spline S145 degree 2 poles (32.2021, 15.4991) (32.2299, 15.6668) (32.2691, 16.1534) (32.2529, 16.474) knots 0 0 0 1 2 2 2
  spline S146 degree 2 poles (32.2529, 16.474) (32.2321, 16.7564) (32.0586, 17.4409) (31.9039, 17.708) knots 0 0 0 1 2 2 2
  spline S147 degree 2 poles (31.9039, 17.708) (31.4358, 18.5162) (29.6447, 18.7901) (28.5293, 18.144) knots 0 0 0 1 2 2 2
  spline S148 degree 2 poles (28.5293, 18.144) (27.4406, 17.5134) (26.7677, 15.8569) (27.2551, 15.0153) knots 0 0 0 1 2 2 2
  spline S149 degree 2 poles (27.2551, 15.0153) (27.5492, 14.5077) (28.5038, 13.8297) (29.0362, 13.6653) knots 0 0 0 1 2 2 2
  line L109 (29.0362, 13.6653) -> (29.071, 13.6052)
  line L110 (29.071, 13.6052) -> (27.9021, 12.9281)
  spline S150 degree 2 poles (27.9021, 12.9281) (27.7397, 13.0392) (27.2618, 13.3868) (27.1067, 13.5467) knots 0 0 0 1 2 2 2
  spline S151 degree 2 poles (27.1067, 13.5467) (26.8718, 13.7675) (26.5479, 14.1419) (26.3584, 14.4691) knots 0 0 0 1 2 2 2
  spline S152 degree 2 poles (28.4026, 9.8227) (28.1707, 10.502) (28.1344, 11.8028) (28.2068, 12.2598) knots 0 0 0 1 2 2 2
  line L111 (28.2068, 12.2598) -> (29.4851, 12.6962)
  line L112 (29.4851, 12.6962) -> (29.5051, 12.6378)
  spline S153 degree 2 poles (29.5051, 12.6378) (29.4381, 12.4518) (29.2952, 11.9625) (29.254, 11.5814) knots 0 0 0 1 2 2 2
  spline S154 degree 2 poles (29.254, 11.5814) (29.2124, 11.2492) (29.2473, 10.4781) (29.3745, 10.1055) knots 0 0 0 1 2 2 2
  spline S155 degree 2 poles (29.3745, 10.1055) (29.4668, 9.8353) (29.8029, 9.2567) (29.9551, 9.1456) knots 0 0 0 1 2 2 2
  spline S156 degree 2 poles (29.9551, 9.1456) (30.1662, 8.9811) (30.5451, 8.8984) (30.8665, 9.0081) knots 0 0 0 1 2 2 2
  spline S157 degree 2 poles (30.8665, 9.0081) (31.2683, 9.1453) (31.535, 9.7257) (31.4818, 10.3356) knots 0 0 0 1 2 2 2
  spline S158 degree 2 poles (31.4818, 10.3356) (31.4581, 10.5722) (31.3648, 11.3233) (31.3429, 11.6503) knots 0 0 0 1 2 2 2
  spline S159 degree 2 poles (31.3429, 11.6503) (31.305, 12.5019) (32.0007, 13.5223) (32.6654, 13.7493) knots 0 0 0 1 2 2 2
  spline S160 degree 2 poles (32.6654, 13.7493) (33.5858, 14.0635) (35.204, 13.0744) (35.593, 11.9348) knots 0 0 0 1 2 2 2
  spline S161 degree 2 poles (35.593, 11.9348) (35.7851, 11.3724) (35.8965, 10.138) (35.8168, 9.6786) knots 0 0 0 1 2 2 2
  line L113 (35.8168, 9.6786) -> (34.5969, 9.2621)
  line L114 (34.5969, 9.2621) -> (34.577, 9.3205)
  spline S162 degree 2 poles (34.577, 9.3205) (34.778, 9.8785) (34.8157, 11.0822) (34.6286, 11.6301) knots 0 0 0 1 2 2 2
  spline S163 degree 2 poles (34.6286, 11.6301) (34.4366, 12.1925) (33.6974, 12.8048) (33.2226, 12.6427) knots 0 0 0 1 2 2 2
  spline S164 degree 2 poles (33.2226, 12.6427) (32.7916, 12.4955) (32.5324, 11.8932) (32.5754, 11.337) knots 0 0 0 1 2 2 2
  spline S165 degree 2 poles (32.5754, 11.337) (32.5945, 11.0661) (32.6775, 10.393) (32.7143, 10.0223) knots 0 0 0 1 2 2 2
  spline S166 degree 2 poles (32.7143, 10.0223) (32.7788, 9.2123) (32.1688, 8.1559) (31.4164, 7.899) knots 0 0 0 1 2 2 2
  spline S167 degree 2 poles (31.4164, 7.899) (30.9781, 7.7494) (30.0866, 7.8284) (29.687, 8.0671) knots 0 0 0 1 2 2 2
  spline S168 degree 2 poles (29.687, 8.0671) (29.2653, 8.3228) (28.6395, 9.1287) (28.4026, 9.8227) knots 0 0 0 1 2 2 2
  point P0 (0, 0)
  point P1 (0, 30.2227)
  dimension "d38" = 3.175
  dimension "d39" = 3.175
  dimension "d40" = 3.175
  dimension "d41" = 19.05
  dimension "d42" = 12.7
  dimension "d43" = 12.7
  dimension "d44" = 12.7
  constraints: 4 end point, 4 point on circle, 3 point on line, 1 centre point, 1 perpendicular, 3 other
  measures "d38" distance between parallel lines of L3 L4
  measures "d39" distance between parallel lines of L5 L1
  measures "d40" distance between parallel lines of L6 L2
  measures "d41" distance between parallel lines of L0 L2
  measures "d42" distance of L5.start A1.start
  measures "d43" distance of L4.end A1.end
  measures "d44" distance of L9.end point (0, 30.223)
extrude "Extrusion9" cut sketch "Sketch11" against normal blind 1.5875 contours L45 L46 L47 L48 | L99 L100 L101 L102 | L76 L69 L9 | L9 L69 L70 L71 L72 L73 L74 L75 S104 S105 S106 L76 | S70 S71 S72 S73 L40 L41 S74 S75 S76 L42 L43 S77 S78 A1 | A1 S78 S70 | S168 S152 A1 | A1 S152 L111 L112 S153 S154 S155 S156 S157 S158 S159 S160 S161 L113 L114 S162 S163 S164 S165 S166 S167 S168 | S112 S113 S114 S111 A1 | A1 S111 S112 | S89 S90 A1 | A1 S90 S91 S92 S93 L62 S94 S95 S96 L63 L64 S97 S98 S99 L65 L66 L67 S88 S89 | S83 L49 L50 L51 L52 L53 L54 L55 L56 L57 L58 L59 S84 S85 S86 L60 L61 S87 A1 | A1 S87 S83 | S151 S140 A1 | A1 S140 S141 S142 S143 S144 L107 L108 S145 S146 S147 S148 S149 L109 L110 S150 S151 | S120 L80 L81 L82 L83 L84 S121 S122 S119 A1 | A1 S119 S120 | S128 S129 S130 S127 A1 | A1 S127 S128 | S139 S135 A1 | A1 S135 L86 L87 L88 L89 L90 L91 L92 L93 L94 L95 L96 S136 S137 S138 L97 L98 S139 | S0 S1 S2 S3 S4 S5 S6 L10 L11 S7 S8 S9 S10 S11 | S19 S20 S21 S22 S23 S24 S25 L12 L13 S26 S27 S28 S29 S30 | L14 L15 L16 L17 | L21 L22 S38 S39 S40 S41 S42 S43 L23 L24 S44 S45 S46 S47 S48 L25 L26 | S49 S50 S51 L27 L28 S52 S53 S54 S55 S56 S57 S58 L29 L30 L31 L32 L33 S59 S60 S61 | S62 S63 L34 L35 L36 S64 S65 | L103 L104 L105 L106
sketch "Sketch12" plane through (-41.275, -25.4, 59.69) normal (0, -1, 0) x (1, 0, 0)
  line L0 (-3.175, -59.69) -> (9.525, -59.69) projected
  line L1 (-3.175, -59.69) -> (-15.5349, -59.69)
  line L2 (-15.5349, -59.69) -> (-15.5349, 3.246)
  line L3 (-15.5349, 3.246) -> (-3.175, 3.246)
  line L4 (-3.175, 3.246) -> (-3.175, -59.69)
  point P0 (41.275, -59.69)
  constraints: 8 end point, 2 parallel, 1 horizontal, 1 perpendicular
extrude "Extrusion10" cut sketch "Sketch12" against normal through all
equation "\"d22\" = d18"
equation "\"d39\" = d38"
equation "\"d40\" = d38"
equation "\"d43\" = d42"
equation "\"d44\" = d42"
body "Solid1"
